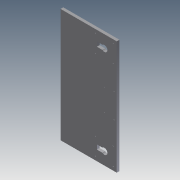
# Autodesk Inventor part: holdertop
Saved by Autodesk Inventor 2011 (Build 150239000, 239)
## iProperties
Created: 2011-09-17
Part Number: holdertop
Document SubType Name: Modeling
Designer: Matthew
Density: 1 g/cm^3
Author: Matthew
Autodesk Inventor part; units mm, degrees
ref_plane "YZ Plane" through (0, 0, 0) normal (1, 0, 0) x (0, 1, 0)
ref_plane "XZ Plane" through (0, 0, 0) normal (0, 1, 0) x (-1, 0, 0)
ref_plane "XY Plane" through (0, 0, 0) normal (0, 0, 1) x (1, 0, 0)
sketch "Sketch1" plane through (0, 0, 0) normal (0, 0, 1) x (1, 0, 0)
  line L0 (-25.4072, 25.3665) -> (76.1928, 25.3665)
  line L1 (76.1928, 25.3665) -> (76.1928, -76.2335)
  line L2 (76.1928, -76.2335) -> (-25.4072, -76.2335)
  line L3 (-25.4072, -76.2335) -> (-25.4072, 25.3665)
  point P0 (0, 0)
  dimension "d0" = 101.6
  dimension "d1" = 101.6
  constraints: 8 end point, 2 parallel, 1 horizontal, 1 perpendicular
  measures "d0" distance of L1.end L2.end
  measures "d1" distance of L0.end L1.end
extrude "Extrusion1" add sketch "Sketch1" along normal blind 0.7366
sketch "Sketch2" plane through (0, 0, 0.7366) normal (0, 0, 1) x (1, 0, 0)
  line L0 (-25.4072, 25.3665) -> (76.1928, -76.2335)
  line L1 (76.1928, 25.3665) -> (-25.4072, -76.2335)
  circle A0 centre (25.3928, -25.4335) radius 27.432
  point P0 (0, 0)
  dimension "d4" = 54.864
  constraints: 4 end point, 1 centre point, 1 midpoint, 1 perpendicular
  measures "d4" diameter of A0
extrude "Extrusion2" cut sketch "Sketch2" against normal blind 0.7366
sketch "Sketch3" plane through (0, 0, 0.7366) normal (0, 0, 1) x (1, 0, 0)
  line L0 (-25.4072, -76.2335) -> (-25.4072, 25.3665) projected
  line L1 (-25.4072, 25.3665) -> (-25.4072, -25.4335)
  line L2 (-25.4072, -25.4335) -> (-25.4072, 19.4102)
  line L3 (-25.4072, 25.3665) -> (76.1928, -76.2335)
  line L4 (76.1928, 25.3665) -> (-25.4072, -76.2335)
  circle A0 centre (-19.4509, 19.4102) radius 1.9812
  point P0 (0, 0)
  dimension "d7" = 44.8437
  dimension "d8" = 3.9624
  constraints: 8 end point, 2 point on line, 1 centre point, 1 midpoint, 1 perpendicular
  measures "d7" distance of L1.end L2.end
  measures "d8" diameter of A0
extrude "Extrusion3" cut sketch "Sketch3" against normal blind 0.7366 contours A0 L3 | L3 A0
sketch "Sketch4" plane through (0, 0, 0.7366) normal (0, 0, 1) x (1, 0, 0)
  line L0 (-25.4072, -76.2335) -> (76.1928, 25.3665)
  line L1 (-25.4072, 25.3665) -> (76.1928, -76.2335)
  circle A0 centre (70.2365, 19.4102) radius 1.9819
  circle A1 centre (70.2365, -70.2772) radius 1.983
  circle A2 centre (-19.4509, -70.2772) radius 1.9812
  point P0 (0, 0)
  constraints: 4 end point, 3 centre point, 3 point on line, 1 perpendicular
extrude "Extrusion4" cut sketch "Sketch4" against normal blind 0.7366
sketch "Sketch5" plane through (0, 0, 0.7366) normal (0, 0, 1) x (1, 0, 0)
  circle A0 centre (25.3928, -25.4335) radius 27.432 projected
  circle A1 centre (25.3928, -25.4335) radius 29.972
  circle A2 centre (25.3928, -25.4335) radius 32.512
  point P0 (0, 0)
  dimension "d13" = 59.944
  dimension "d14" = 65.024
  constraints: 2 centre point, 2 coincident
  measures "d13" diameter of A1
  measures "d14" diameter of A2
extrude "Extrusion5" add sketch "Sketch5" along normal blind 6.6548 contours A2
fillet "Fillet1" radius 3.175 4 edges at (-25.4072, 25.3665, 0.3683) (76.1928, 25.3665, 0.3683) (76.1928, -76.2335, 0.3683) (-25.4072, -76.2335, 0.3683)
sketch "Sketch6" plane through (25.3928, -25.4335, 0.7366) normal (0, 0, 1) x (1, 0, 0)
  circle A0 centre (0, 0) radius 29.972 projected
  circle A1 centre (0, 0) radius 27.432 projected
  point P0 (-25.3928, 25.4335)
extrude "Extrusion6" add sketch "Sketch6" along normal blind 9.1948
sketch "Sketch7" plane through (25.3928, -25.4335, 7.3914) normal (0, 0, 1) x (1, 0, 0)
  circle A0 centre (0, 0) radius 29.972 projected
  circle A1 centre (0, 0) radius 32.512 projected
  point P0 (-25.3928, 25.4335)
extrude "Extrusion7" cut sketch "Sketch7" against normal blind 6.6548
sketch "Sketch8" plane through (25.3928, -25.4335, 9.9314) normal (0, 0, 1) x (1, 0, 0)
  circle A0 centre (0, 0) radius 27.432 projected
  circle A1 centre (0, 0) radius 29.972 projected
  point P0 (-25.3928, 25.4335)
extrude "Extrusion8" cut sketch "Sketch8" against normal blind 2.54
sketch "Sketch9" plane through (0, 0, 0.7366) normal (0, 0, 1) x (1, 0, 0)
  circle A0 centre (-19.4509, 19.4102) radius 1.9812 projected
  circle A1 centre (70.2365, -70.2772) radius 1.983 projected
  circle A2 centre (-19.4509, -70.2772) radius 1.9812 projected
  circle A3 centre (70.2365, 19.4102) radius 1.9819 projected
  point P0 (0, 0)
extrude "Extrusion9" add sketch "Sketch9" against normal blind 0.7366
sketch "Sketch10" plane through (0, 0, 0.7366) normal (0, 0, 1) x (1, 0, 0)
  line L0 (-25.4072, 25.3665) -> (76.1928, 25.3665)
  line L1 (76.1928, 25.3665) -> (76.1928, -76.2335)
  line L2 (76.1928, -76.2335) -> (-25.4072, -76.2335)
  line L3 (-25.4072, -76.2335) -> (-25.4072, 25.3665)
  line L4 (-25.4072, 25.3665) -> (76.1928, -76.2335)
  line L5 (-25.4072, -76.2335) -> (76.1928, 25.3665)
  line L6 (-25.4072, 25.3665) -> (-25.4072, -25.4335)
  line L7 (-25.4072, -25.4335) -> (-25.4072, 15.0541)
  circle A0 centre (-15.0948, 15.0541) radius 1.9812
  circle A1 centre (65.8804, 15.0541) radius 1.9818
  circle A2 centre (65.8804, -65.9211) radius 1.9832
  circle A3 centre (-15.0948, -65.9211) radius 1.9812
  point P0 (0, 0)
  dimension "d26" = 40.4876
  dimension "d27" = 3.9624
  constraints: 16 end point, 5 point on line, 4 centre point, 2 parallel, 2 perpendicular, 1 horizontal, 1 midpoint
  measures "d26" distance of L6.end L7.end
  measures "d27" diameter of A0
extrude "Extrusion10" cut sketch "Sketch10" against normal blind 0.7366 contours A0 L4 | L4 A0 | A1 L5 | L5 A1 | A2 L4 | L4 A2 | A3 L5 | L5 A3
sketch "Sketch11" plane through (0, 0, 0.7366) normal (0, 0, 1) x (1, 0, 0)
  circle A0 centre (-15.0948, 15.0541) radius 1.9812 projected
  circle A1 centre (-15.0948, -65.9211) radius 1.9812 projected
  circle A2 centre (65.8804, 15.0541) radius 1.9818 projected
  circle A3 centre (65.8804, -65.9211) radius 1.9832 projected
  line L0 (-25.4072, 25.3665) -> (76.1928, 25.3665)
  line L1 (76.1928, 25.3665) -> (76.1928, -76.2335)
  line L2 (76.1928, -76.2335) -> (-25.4072, -76.2335)
  line L3 (-25.4072, -76.2335) -> (-25.4072, 25.3665)
  point P0 (0, 0)
  constraints: 8 end point, 2 parallel, 1 horizontal, 1 perpendicular
extrude "Extrusion11" add sketch "Sketch11" along normal blind 12.7
sketch "Sketch12" plane through (0, 0, 13.4366) normal (0, 0, 1) x (1, 0, 0)
  circle A0 centre (65.8804, -65.9211) radius 1.9832 projected
  circle A1 centre (65.8804, 15.0541) radius 1.9818 projected
  circle A2 centre (-15.0948, 15.0541) radius 1.9812 projected
  circle A3 centre (-15.0948, -65.9211) radius 1.9812 projected
  line L0 (76.1928, 25.3665) -> (76.1928, -76.2335) projected
  line L1 (-25.4072, 25.3665) -> (76.1928, 25.3665) projected
  line L2 (-25.4072, -76.2335) -> (-25.4072, 25.3665) projected
  line L3 (76.1928, -76.2335) -> (-25.4072, -76.2335) projected
  point P0 (0, 0)
extrude "Extrusion12" add sketch "Sketch12" against normal blind 19.05
sketch "Sketch13" plane through (0, 0, 13.4366) normal (0, 0, 1) x (1, 0, 0)
  circle A0 centre (65.8804, -65.9211) radius 1.9832 projected
  circle A1 centre (65.8804, 15.0541) radius 1.9818 projected
  circle A2 centre (-15.0948, 15.0541) radius 1.9812 projected
  circle A3 centre (-15.0948, -65.9211) radius 1.9812 projected
  line L0 (76.1928, 25.3665) -> (76.1928, -76.2335) projected
  line L1 (-25.4072, 25.3665) -> (76.1928, 25.3665) projected
  line L2 (-25.4072, -76.2335) -> (-25.4072, 25.3665) projected
  line L3 (76.1928, -76.2335) -> (-25.4072, -76.2335) projected
  point P0 (0, 0)
extrude "Extrusion13" cut sketch "Sketch13" against normal blind 12.7
sketch "Sketch14" plane through (-25.4072, 25.3665, -5.6134) normal (0, 1, 0) x (1, 0, 0)
  line L0 (0, -6.35) -> (101.6, -6.35) projected
  line L1 (101.6, -6.35) -> (101.6, 0) projected
  line L2 (101.6, 0) -> (0, 0) projected
  line L3 (0, 0) -> (0, -6.35) projected
  point P0 (25.4072, -5.6134)
sketch "Sketch15" plane through (-25.4072, -76.2335, -5.6134) normal (-1, 0, 0) x (0, 0, 1)
  line L0 (6.35, 0) -> (6.35, 101.6) projected
  line L1 (0, 101.6) -> (6.35, 101.6) projected
  line L2 (0, 101.6) -> (0, 0) projected
  line L3 (6.35, 0) -> (0, 0) projected
  point P0 (5.6134, 76.2335)
sketch "Sketch16" plane through (-25.4072, -76.2335, -5.6134) normal (0, -1, 0) x (1, 0, 0)
  line L0 (101.6, 6.35) -> (0, 6.35) projected
  line L1 (0, 6.35) -> (0, 0) projected
  line L2 (0, 0) -> (101.6, 0) projected
  line L3 (101.6, 6.35) -> (101.6, 0) projected
  point P0 (25.4072, 5.6134)
sketch "Sketch17" plane through (76.1928, -76.2335, -5.6134) normal (1, 0, 0) x (0, 0, -1)
  line L0 (-6.35, 101.6) -> (-6.35, 0) projected
  line L1 (-6.35, 0) -> (0, 0) projected
  line L2 (0, 0) -> (0, 101.6) projected
  line L3 (-6.35, 101.6) -> (0, 101.6) projected
  point P0 (-5.6134, 76.2335)
extrude "Extrusion14" add sketch "Sketch14" along normal blind 53.975
extrude "Extrusion15" add sketch "Sketch17" along normal blind 47.625
extrude "Extrusion16" add sketch "Sketch16" along normal blind 47.625
extrude "Extrusion17" add sketch "Sketch15" along normal blind 53.975
sketch "Sketch18" plane through (-25.4072, 25.3665, 0.7366) normal (0, 1, 0) x (1, 0, 0)
  line L0 (-53.975, 6.35) -> (-53.975, 0) projected
  line L1 (0, 0) -> (-53.975, 0) projected
  line L2 (0, 6.35) -> (0, 0) projected
  line L3 (0, 6.35) -> (-53.975, 6.35) projected
  point P0 (25.4072, 0.7366)
extrude "Extrusion18" add sketch "Sketch18" along normal blind 53.975
sketch "Sketch19" plane through (76.1928, 25.3665, 0.7366) normal (0, 1, 0) x (1, 0, 0)
  line L0 (47.625, 0) -> (47.625, 6.35) projected
  line L1 (0, 6.35) -> (47.625, 6.35) projected
  line L2 (0, 0) -> (0, 6.35) projected
  line L3 (0, 0) -> (47.625, 0) projected
  point P0 (-76.1928, 0.7366)
extrude "Extrusion19" add sketch "Sketch19" along normal blind 53.975
sketch "Sketch20" plane through (-25.4072, -123.8585, -5.6134) normal (-1, 0, 0) x (0, 0, 1)
  line L0 (6.35, 47.625) -> (0, 47.625) projected
  line L1 (0, 47.625) -> (0, 0) projected
  line L2 (0, 0) -> (6.35, 0) projected
  line L3 (6.35, 0) -> (6.35, 47.625) projected
  point P0 (5.6134, 123.8585)
extrude "Extrusion20" add sketch "Sketch20" along normal blind 53.975
sketch "Sketch21" plane through (123.8178, -76.2335, -5.6134) normal (0, -1, 0) x (1, 0, 0)
  line L0 (-47.625, 6.35) -> (-47.625, 0) projected
  line L1 (-47.625, 0) -> (0, 0) projected
  line L2 (0, 0) -> (0, 6.35) projected
  line L3 (0, 6.35) -> (-47.625, 6.35) projected
  point P0 (-123.8178, 5.6134)
extrude "Extrusion21" add sketch "Sketch21" along normal blind 47.625
sketch "Sketch22" plane through (-25.4072, 79.3415, -5.6134) normal (0, 1, 0) x (1, 0, 0)
  line L0 (149.225, -6.35) -> (-53.975, -6.35) projected
  line L1 (149.225, 0) -> (149.225, -6.35) projected
  line L2 (-53.975, 0) -> (149.225, 0) projected
  line L3 (-53.975, -6.35) -> (-53.975, 0) projected
  point P0 (25.4072, -5.6134)
extrude "Extrusion22" cut sketch "Sketch22" against normal blind 53.975
sketch "Sketch23" plane through (-79.3822, -76.2335, -5.6134) normal (-1, 0, 0) x (0, 0, 1)
  line L0 (6.35, 101.6) -> (0, 101.6) projected
  line L1 (0, -47.625) -> (0, 101.6) projected
  line L2 (6.35, -47.625) -> (0, -47.625) projected
  line L3 (6.35, 101.6) -> (6.35, -47.625) projected
  point P0 (5.6134, 76.2335)
extrude "Extrusion23" cut sketch "Sketch23" against normal blind 53.975
sketch "Sketch24" plane through (-25.4072, -123.8585, -5.6134) normal (0, -1, 0) x (1, 0, 0)
  line L0 (0, 6.35) -> (0, 0) projected
  line L1 (149.225, 0) -> (0, 0) projected
  line L2 (149.225, 6.35) -> (149.225, 0) projected
  line L3 (0, 6.35) -> (149.225, 6.35) projected
  point P0 (25.4072, 5.6134)
extrude "Extrusion24" cut sketch "Sketch24" against normal blind 47.625
sketch "Sketch25" plane through (123.8178, -76.2335, -5.6134) normal (1, 0, 0) x (0, 0, -1)
  line L0 (-6.35, 0) -> (0, 0) projected
  line L1 (0, 101.6) -> (0, 0) projected
  line L2 (0, 101.6) -> (-6.35, 101.6) projected
  line L3 (-6.35, 0) -> (-6.35, 101.6) projected
  point P0 (-5.6134, 76.2335)
extrude "Extrusion25" cut sketch "Sketch25" against normal blind 47.625
sketch "Sketch26" plane through (-25.4072, 25.3665, -5.6134) normal (0, 1, 0) x (1, 0, 0)
  line L0 (101.6, -6.35) -> (101.6, 0) projected
  line L1 (0, 0) -> (101.6, 0) projected
  line L2 (0, 0) -> (0, -6.35) projected
  line L3 (101.6, -6.35) -> (0, -6.35) projected
  point P0 (25.4072, -5.6134)
extrude "Extrusion26" add sketch "Sketch26" along normal blind 53.975
sketch "Sketch27" plane through (-25.4072, -76.2335, -5.6134) normal (-1, 0, 0) x (0, 0, 1)
  line L0 (0, 0) -> (6.35, 0) projected
  line L1 (6.35, 0) -> (6.35, 155.575) projected
  line L2 (6.35, 155.575) -> (0, 155.575) projected
  line L3 (0, 0) -> (0, 155.575) projected
  point P0 (5.6134, 76.2335)
extrude "Extrusion27" add sketch "Sketch27" along normal blind 53.975
sketch "Sketch28" plane through (-25.4072, -76.2335, -5.6134) normal (0, -1, 0) x (1, 0, 0)
  line L0 (101.6, 0) -> (101.6, 6.35) projected
  line L1 (101.6, 6.35) -> (-53.975, 6.35) projected
  line L2 (-53.975, 6.35) -> (-53.975, 0) projected
  line L3 (101.6, 0) -> (-53.975, 0) projected
  point P0 (25.4072, 5.6134)
extrude "Extrusion28" add sketch "Sketch28" along normal blind 22.225
sketch "Sketch29" plane through (-25.4072, 79.3415, -5.6134) normal (0, 1, 0) x (1, 0, 0)
  line L0 (101.6, -6.35) -> (-53.975, -6.35) projected
  line L1 (101.6, 0) -> (101.6, -6.35) projected
  line L2 (-53.975, 0) -> (101.6, 0) projected
  line L3 (-53.975, 0) -> (-53.975, -6.35) projected
  point P0 (25.4072, -5.6134)
extrude "Extrusion29" add sketch "Sketch29" along normal blind 158.6992
sketch "Sketch30" plane through (-25.4072, 238.0407, -5.6134) normal (0, 1, 0) x (1, 0, 0)
  line L0 (-53.975, -6.35) -> (-53.975, 0) projected
  line L1 (101.6, -6.35) -> (-53.975, -6.35) projected
  line L2 (101.6, 0) -> (101.6, -6.35) projected
  line L3 (-53.975, 0) -> (101.6, 0) projected
  point P0 (25.4072, -5.6134)
extrude "Extrusion30" add sketch "Sketch30" along normal blind 177.8
sketch "Sketch31" plane through (0, 0, 0.7366) normal (0, 0, 1) x (1, 0, 0)
  line L0 (76.1928, 415.8407) -> (76.1928, -98.4585) projected
  line L1 (76.1928, 415.8407) -> (-79.3822, 415.8407) projected
  line L2 (65.8804, 415.8407) -> (65.8804, 383.3033)
  line L3 (65.8804, 383.3033) -> (-17.076, 383.3033)
  line L4 (-17.076, 383.3033) -> (-13.1136, 383.3033)
  line L5 (-13.1136, 383.3033) -> (-15.0948, 383.3033)
  circle A0 centre (-15.0948, 383.3033) radius 1.9812
  circle A1 centre (65.8804, 383.3033) radius 1.9812
  line L6 (65.8804, 383.3033) -> (65.8804, 302.3281)
  circle A2 centre (65.8804, 302.3281) radius 1.9812
  line L7 (-15.0948, 383.3033) -> (-15.0948, 302.3281)
  circle A3 centre (-15.0948, 302.3281) radius 1.9812
  point P0 (0, 0)
  dimension "d70" = 32.5374
  dimension "d71" = 80.9752
  constraints: 12 end point, 4 coincident, 3 centre point, 2 parallel, 2 perpendicular, 2 point on line, 1 horizontal alignment, 1 midpoint, 2 other
  measures "d70" distance of L2.start L2.end
  measures "d71" distance of L6.start L6.end
extrude "Extrusion31" cut sketch "Sketch31" against normal blind 177.8
sketch "Sketch32" plane through (0, 0, -5.6134) normal (0, 0, -1) x (-1, 0, 0)
  circle A0 centre (15.0948, 383.3033) radius 1.9812 projected
  circle A1 centre (15.0948, 302.3281) radius 1.9812 projected
  circle A2 centre (-65.8804, 302.3281) radius 1.9812 projected
  circle A3 centre (-65.8804, 383.3033) radius 1.9812 projected
  circle A4 centre (15.0948, -65.9211) radius 1.9812 projected
  circle A5 centre (15.0948, 15.0541) radius 1.9812 projected
  circle A6 centre (-65.8804, 15.0541) radius 1.9818 projected
  circle A7 centre (-65.8804, -65.9211) radius 1.9832 projected
  line L0 (-76.1928, 415.8407) -> (-76.1928, -98.4585) projected
  line L1 (-76.1928, -98.4585) -> (79.3822, -98.4585) projected
  line L2 (79.3822, -98.4585) -> (79.3822, 415.8407) projected
  line L3 (79.3822, 415.8407) -> (-76.1928, 415.8407) projected
  point P0 (0, 0)
extrude "Extrusion32" add sketch "Sketch32" along normal blind 6.35
sketch "Sketch33" plane through (-79.3822, -76.2335, -5.6134) normal (-1, 0, 0) x (0, 0, 1)
  line L0 (-6.35, -22.225) -> (6.35, -22.225) projected
  line L1 (6.35, 492.0742) -> (6.35, -22.225) projected
  line L2 (6.35, 492.0742) -> (-6.35, 492.0742) projected
  line L3 (-6.35, 492.0742) -> (-6.35, -22.225) projected
  point P0 (5.6134, 76.2335)
extrude "Extrusion33" add sketch "Sketch33" along normal blind 6.35
sketch "Sketch34" plane through (-25.4072, 415.8407, -5.6134) normal (0, 1, 0) x (1, 0, 0)
  line L0 (101.6, -6.35) -> (-60.325, -6.35) projected
  line L1 (101.6, 6.35) -> (101.6, -6.35) projected
  line L2 (101.6, 6.35) -> (-60.325, 6.35) projected
  line L3 (-60.325, 6.35) -> (-60.325, -6.35) projected
  point P0 (25.4072, -5.6134)
extrude "Extrusion34" add sketch "Sketch34" along normal blind 6.35
sketch "Sketch35" plane through (-25.4072, -98.4585, -5.6134) normal (0, -1, 0) x (1, 0, 0)
  line L0 (101.6, 6.35) -> (101.6, -6.35) projected
  line L1 (-60.325, 6.35) -> (101.6, 6.35) projected
  line L2 (-60.325, 6.35) -> (-60.325, -6.35) projected
  line L3 (-60.325, -6.35) -> (101.6, -6.35) projected
  point P0 (25.4072, 5.6134)
extrude "Extrusion35" add sketch "Sketch35" along normal blind 6.35
sketch "Sketch36" plane through (-85.7322, -76.2335, -5.6134) normal (-1, 0, 0) x (0, 0, 1)
  line L0 (-6.35, -28.575) -> (-6.35, 498.4242) projected
  line L1 (-6.35, -28.575) -> (6.35, -28.575) projected
  line L2 (6.35, 498.4242) -> (6.35, -28.575) projected
  line L3 (6.35, 498.4242) -> (-6.35, 498.4242) projected
  point P0 (5.6134, 76.2335)
extrude "Extrusion36" cut sketch "Sketch36" against normal blind 6.35
sketch "Sketch37" plane through (76.1928, -76.2335, -5.6134) normal (1, 0, 0) x (0, 0, -1)
  line L0 (-6.35, 498.4242) -> (-6.35, -28.575) projected
  line L1 (-6.35, -28.575) -> (6.35, -28.575) projected
  line L2 (6.35, -28.575) -> (6.35, 498.4242) projected
  line L3 (6.35, 498.4242) -> (-6.35, 498.4242) projected
  point P0 (-5.6134, 76.2335)
extrude "Extrusion37" add sketch "Sketch37" along normal blind 6.35
sketch "Sketch38" plane through (-79.3822, -76.2335, -5.6134) normal (-1, 0, 0) x (0, 0, 1)
  line L0 (6.35, -28.575) -> (-6.35, -28.575) projected
  line L1 (6.35, 498.4242) -> (6.35, -28.575) projected
  line L2 (-6.35, 498.4242) -> (6.35, 498.4242) projected
  line L3 (-6.35, -28.575) -> (-6.35, 498.4242) projected
  point P0 (5.6134, 76.2335)
extrude "Extrusion38" add sketch "Sketch38" along normal blind 98.425
sketch "Sketch39" plane through (0, 0, -11.9634) normal (0, 0, -1) x (-1, 0, 0)
  line L0 (177.8072, 422.1907) -> (-82.5428, 422.1907) projected
  line L1 (-82.5428, 422.1907) -> (-82.5428, -104.8085) projected
  line L2 (-82.5428, -104.8085) -> (177.8072, -104.8085) projected
  line L3 (177.8072, -104.8085) -> (177.8072, 422.1907) projected
  circle A0 centre (15.0948, 302.3281) radius 1.9812 projected
  circle A1 centre (-65.8804, 302.3281) radius 1.9812 projected
  circle A2 centre (-65.8804, 383.3033) radius 1.9812 projected
  circle A3 centre (15.0948, -65.9211) radius 1.9812 projected
  circle A4 centre (15.0948, 383.3033) radius 1.9812 projected
  circle A5 centre (15.0948, 15.0541) radius 1.9812 projected
  circle A6 centre (-65.8804, 15.0541) radius 1.9818 projected
  circle A7 centre (-65.8804, -65.9211) radius 1.9832 projected
  point P0 (0, 0)
extrude "Extrusion39" cut sketch "Sketch39" against normal blind 6.35
sketch "Sketch40" plane through (0, 0, -5.6134) normal (0, 0, -1) x (-1, 0, 0)
  circle A0 centre (-65.8804, -65.9211) radius 1.9832 projected
  circle A1 centre (-65.8804, 15.0541) radius 1.9818 projected
  circle A2 centre (15.0948, 15.0541) radius 1.9812 projected
  circle A3 centre (15.0948, 383.3033) radius 1.9812 projected
  circle A4 centre (15.0948, -65.9211) radius 1.9812 projected
  circle A5 centre (-65.8804, 383.3033) radius 1.9812 projected
  circle A6 centre (-65.8804, 302.3281) radius 1.9812 projected
  circle A7 centre (15.0948, 302.3281) radius 1.9812 projected
  line L0 (-82.5428, -104.8085) -> (-82.5428, 422.1907) projected
  line L1 (177.8072, -104.8085) -> (-82.5428, -104.8085) projected
  line L2 (177.8072, 422.1907) -> (177.8072, -104.8085) projected
  line L3 (-82.5428, 422.1907) -> (177.8072, 422.1907) projected
  point P0 (0, 0)
extrude "Extrusion40" add sketch "Sketch40" along normal blind 6.35
sketch "Sketch41" plane through (0, 0, -11.9634) normal (0, 0, -1) x (-1, 0, 0)
  circle A0 centre (-65.8804, -65.9211) radius 1.9832 projected
  circle A1 centre (15.0948, 15.0541) radius 1.9812 projected
  circle A2 centre (15.0948, 383.3033) radius 1.9812 projected
  circle A3 centre (15.0948, 302.3281) radius 1.9812 projected
  line L0 (177.8072, 422.1907) -> (177.8072, -104.8085) projected
  line L1 (15.0948, 15.0541) -> (15.0948, -7.1709)
  line L2 (15.0948, -7.1709) -> (-65.8804, -7.1709)
  line L3 (-65.8804, -65.9211) -> (-65.8804, -88.1461)
  line L4 (-65.8804, -88.1461) -> (15.0948, -88.1461)
  circle A4 centre (15.0948, -7.1709) radius 1.9812
  circle A5 centre (-65.8804, -7.1709) radius 1.9812
  circle A6 centre (-65.8804, -88.1461) radius 1.9812
  circle A7 centre (15.0948, -88.1461) radius 1.9812
  line L5 (15.0948, 383.3033) -> (15.0948, 405.5283)
  line L6 (15.0948, 405.5283) -> (-65.8804, 405.5283)
  line L7 (15.0948, 302.3281) -> (15.0948, 324.5531)
  line L8 (15.0948, 324.5531) -> (-65.8804, 324.5531)
  circle A8 centre (15.0948, 405.5283) radius 1.9812
  circle A9 centre (-65.8804, 405.5283) radius 1.9812
  circle A10 centre (-65.8804, 324.5531) radius 1.9812
  circle A11 centre (15.0948, 324.5531) radius 1.9812
  point P0 (0, 0)
  dimension "d92" = 22.225
  dimension "d93" = 22.225
  dimension "d94" = 22.225
  dimension "d95" = 22.225
  constraints: 16 end point, 8 centre point, 8 coincident, 7 perpendicular, 1 parallel
  measures "d92" distance of L1.start L1.end
  measures "d93" distance of L3.start L3.end
  measures "d94" distance of L5.start L5.end
  measures "d95" distance of L7.start L7.end
extrude "Extrusion41" cut sketch "Sketch41" against normal blind 25.4 contours A4 L2 L1 | L1 L2 A4 | A6 L4 L3 | L3 L4 A6 | A5 | A7 | A8 L6 L5 | L5 L6 A8 | A11 L8 L7 | L7 L8 A11 | A9 | A10
sketch "Sketch42" plane through (0, 0, -11.9634) normal (0, 0, -1) x (-1, 0, 0)
  circle A0 centre (-65.8804, -65.9211) radius 1.9832 projected
  circle A1 centre (-65.8804, 15.0541) radius 1.9818 projected
  circle A2 centre (15.0948, 15.0541) radius 1.9812 projected
  circle A3 centre (15.0948, 383.3033) radius 1.9812 projected
  circle A4 centre (15.0948, -65.9211) radius 1.9812 projected
  circle A5 centre (15.0948, 302.3281) radius 1.9812 projected
  circle A6 centre (-65.8804, 302.3281) radius 1.9812 projected
  circle A7 centre (-65.8804, 383.3033) radius 1.9812 projected
  point P0 (0, 0)
extrude "Extrusion42" add sketch "Sketch42" against normal blind 6.35
sketch "Sketch43" plane through (0, 0, 0.7366) normal (0, 0, 1) x (1, 0, 0)
  circle A0 centre (-15.0948, 324.5531) radius 1.9812 projected
  circle A1 centre (65.8804, 324.5531) radius 1.9812 projected
  circle A2 centre (65.8804, 405.5283) radius 1.9812 projected
  circle A3 centre (-15.0948, 405.5283) radius 1.9812 projected
  circle A4 centre (-15.0948, -88.1461) radius 1.9812 projected
  circle A5 centre (65.8804, -88.1461) radius 1.9812 projected
  circle A6 centre (65.8804, -7.1709) radius 1.9812 projected
  circle A7 centre (-15.0948, -7.1709) radius 1.9812 projected
  line L0 (-177.8072, -104.8085) -> (82.5428, -104.8085) projected
  line L1 (82.5428, -104.8085) -> (82.5428, 422.1907) projected
  line L2 (82.5428, 422.1907) -> (-177.8072, 422.1907) projected
  line L3 (-177.8072, 422.1907) -> (-177.8072, -104.8085) projected
  point P0 (0, 0)
extrude "Extrusion43" add sketch "Sketch43" against normal blind 12.7
sketch "Sketch44" plane through (0, 0, -11.9634) normal (0, 0, -1) x (-1, 0, 0)
  circle A0 centre (15.0948, 324.5531) radius 1.9812 projected
  circle A1 centre (-65.8804, 405.5283) radius 1.9812 projected
  circle A2 centre (15.0948, 405.5283) radius 1.9812 projected
  circle A3 centre (15.0948, -88.1461) radius 1.9812 projected
  circle A4 centre (-65.8804, -88.1461) radius 1.9812 projected
  circle A5 centre (15.0948, -7.1709) radius 1.9812 projected
  line L0 (177.8072, 422.1907) -> (177.8072, -104.8085) projected
  line L1 (-65.8804, -88.1461) -> (15.0948, -88.1461)
  line L2 (15.0948, -7.1709) -> (15.0948, -88.1461)
  circle A6 centre (-25.3928, -47.6585) radius 11.25
  line L3 (-25.3928, -47.6585) -> (-25.3928, -37.1585)
  line L4 (-25.3928, -37.1585) -> (9.6072, -37.1585)
  line L5 (9.6072, -37.1585) -> (9.6072, -58.1585)
  line L6 (9.6072, -58.1585) -> (-25.3928, -58.1585)
  line L7 (-25.3928, -58.1585) -> (-25.3928, -37.1585)
  line L8 (15.0948, 324.5531) -> (15.0948, 405.5283)
  line L9 (15.0948, 405.5283) -> (-65.8804, 405.5283)
  circle A7 centre (-25.3928, 365.0407) radius 11.25
  line L10 (-25.3928, 365.0407) -> (-25.3928, 375.5407)
  line L11 (-25.3928, 375.5407) -> (9.6072, 375.5407)
  line L12 (9.6072, 375.5407) -> (9.6072, 354.5407)
  line L13 (9.6072, 354.5407) -> (-25.3928, 354.5407)
  line L14 (-25.3928, 354.5407) -> (-25.3928, 375.5407)
  circle A8 centre (-25.3928, 365.0407) radius 11.5
  circle A9 centre (-25.3928, -47.6585) radius 11.5
  point P0 (0, 0)
  dimension "d102" = 22.5
  dimension "d103" = 10.5
  dimension "d104" = 35
  dimension "d105" = 21
  dimension "d106" = 10.5
  dimension "d107" = 21
  dimension "d108" = 23
  dimension "d109" = 23
  constraints: 28 end point, 6 parallel, 6 perpendicular, 4 centre point, 2 coincident, 2 horizontal
  measures "d102" diameter of A6
  measures "d103" distance of L3.start L3.end
  measures "d104" distance of L5.end L6.end
  measures "d105" distance of L4.end L5.end
  measures "d106" distance of L10.start L10.end
  measures "d107" distance of L11.end L12.end
  measures "d108" diameter of A8
  measures "d109" diameter of A9
extrude "Extrusion44" cut sketch "Sketch44" against normal blind 12.7 contours A6 L6 L7 L3 L4 | A6 L4 A9 L6 | L4 L3 L7 L6 A6 | A6 L6 A9 L4 | L4 L5 L6 A9 | A7 L13 L14 L10 L11 | A7 L11 A8 L13 | L11 L10 L14 L13 A7 | A7 L13 A8 L11 | L11 L12 L13 A8
sketch "Sketch45" plane through (0, 0, -11.9634) normal (0, 0, -1) x (-1, 0, 0)
  arc A0 (-20.7024, -37.1585) -> (-20.7024, -58.1585) centre (-25.3928, -47.6585) ccw projected
  line L0 (-20.7024, 375.5407) -> (9.6072, 375.5407) projected
  line L1 (9.6072, 375.5407) -> (9.6072, 354.5407) projected
  line L2 (9.6072, 354.5407) -> (-20.7024, 354.5407) projected
  arc A1 (-20.7024, 375.5407) -> (-20.7024, 354.5407) centre (-25.3928, 365.0407) ccw projected
  circle A2 centre (-25.3928, 365.0407) radius 14
  circle A3 centre (-25.3928, -47.6585) radius 14
  point P0 (0, 0)
  dimension "d112" = 28
  dimension "d113" = 28
  constraints: 2 centre point, 2 coincident
  measures "d112" diameter of A2
  measures "d113" diameter of A3
extrude "Extrusion45" cut sketch "Sketch45" against normal blind 25.4
sketch "Sketch46" plane through (0, 0, -11.9634) normal (0, 0, -1) x (-1, 0, 0)
  line L0 (-82.5428, -104.8085) -> (-82.5428, 422.1907) projected
  line L1 (-82.5428, 158.6911) -> (-82.5428, 228.5411)
  line L2 (-82.5428, 228.5411) -> (-6.3428, 228.5411)
  line L3 (-6.3428, 228.5411) -> (-6.3428, 88.8411)
  line L4 (-6.3428, 88.8411) -> (-82.5428, 88.8411)
  line L5 (-82.5428, 88.8411) -> (-82.5428, 228.5411)
  line L6 (-82.5428, 228.5411) -> (-69.8428, 228.5411)
  line L7 (-69.8428, 228.5411) -> (-69.8428, 215.8411)
  line L8 (-69.8428, 215.8411) -> (-82.5428, 215.8411)
  line L9 (-82.5428, 215.8411) -> (-82.5428, 228.5411)
  line L10 (-82.5428, 88.8411) -> (-69.8428, 88.8411)
  line L11 (-69.8428, 88.8411) -> (-69.8428, 101.5411)
  line L12 (-69.8428, 101.5411) -> (-82.5428, 101.5411)
  line L13 (-82.5428, 101.5411) -> (-82.5428, 88.8411)
  line L14 (-6.3428, 228.5411) -> (-25.3928, 228.5411)
  line L15 (-25.3928, 228.5411) -> (-25.3928, 209.4911)
  line L16 (-25.3928, 209.4911) -> (-6.3428, 209.4911)
  line L17 (-6.3428, 209.4911) -> (-6.3428, 228.5411)
  line L18 (-6.3428, 88.8411) -> (-25.3928, 88.8411)
  line L19 (-25.3928, 88.8411) -> (-25.3928, 107.8911)
  line L20 (-25.3928, 107.8911) -> (-6.3428, 107.8911)
  line L21 (-6.3428, 107.8911) -> (-6.3428, 88.8411)
  circle A0 centre (-25.3928, 209.4911) radius 1.9812
  circle A1 centre (-69.8428, 215.8411) radius 1.9812
  circle A2 centre (-69.8428, 101.5411) radius 1.9812
  circle A3 centre (-25.3928, 107.8911) radius 1.9812
  point P0 (0, 0)
  dimension "d116" = 69.85
  dimension "d117" = 76.2
  dimension "d118" = 139.7
  dimension "d119" = 12.7
  dimension "d120" = 12.7
  dimension "d121" = 12.7
  dimension "d122" = 12.7
  dimension "d123" = 19.05
  dimension "d124" = 19.05
  dimension "d125" = 19.05
  dimension "d126" = 19.05
  dimension "d127" = 3.9624
  dimension "d128" = 3.9624
  constraints: 42 end point, 10 parallel, 5 horizontal, 5 perpendicular, 4 centre point, 4 coincident, 1 midpoint, 1 point on line
  measures "d116" distance of L1.start L1.end
  measures "d117" distance of L3.end L4.end
  measures "d118" distance of L2.end L3.end
  measures "d119" distance of L7.end L8.end
  measures "d120" distance of L6.end L7.end
  measures "d121" distance of L12.end L11.end
  measures "d122" distance of L11.end L10.end
  measures "d123" distance of L16.end L15.end
  measures "d124" distance of L15.end L14.end
  measures "d125" distance of L19.end L20.end
  measures "d126" distance of L18.end L19.end
  measures "d127" diameter of A0
  measures "d128" diameter of A1
extrude "Extrusion46" cut sketch "Sketch46" against normal blind 25.4 contours A2 L11 L12 | L12 L11 A2 | A3 L20 L19 | L19 L20 A3 | A1 L7 L8 | L8 L7 A1 | A0 L15 L16 | L16 L15 A0
sketch "Sketch47" plane through (0, 0, -11.9634) normal (0, 0, -1) x (-1, 0, 0)
  line L0 (-82.5428, -104.8085) -> (-82.5428, 422.1907) projected
  line L1 (177.8072, 422.1907) -> (177.8072, -104.8085) projected
  line L2 (-82.5428, 158.6911) -> (44.4572, 158.6911)
  circle A0 centre (44.4572, 158.6911) radius 12.7
  point P0 (0, 0)
  dimension "d131" = 127
  dimension "d132" = 25.4
  constraints: 2 end point, 1 centre point, 1 coincident, 1 midpoint, 1 perpendicular
  measures "d131" distance of L2.start L2.end
  measures "d132" diameter of A0
extrude "Extrusion47" cut sketch "Sketch47" against normal blind 25.4
body "Solid1"
